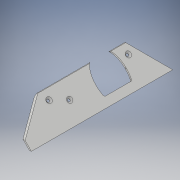
# Autodesk Inventor part: Bok2mm
Saved by Autodesk Inventor 2019 (Build 230136000, 136)
## iProperties
Created: 2022-01-23
Part Number: Bok2mm
Material: Ogólny
Document SubType Name: Modeling
Designer: Michał
Density: 1 g/cm^3
Appearance: Domyślna
Author: Michał
Autodesk Inventor part; units mm, degrees
ref_plane "YZ Plane" through (0, 0, 0) normal (1, 0, 0) x (0, 1, 0)
ref_plane "XZ Plane" through (0, 0, 0) normal (0, 1, 0) x (-1, 0, 0)
ref_plane "XY Plane" through (0, 0, 0) normal (0, 0, 1) x (1, 0, 0)
sketch "Szkic1" plane through (0, 0, 0) normal (0, 0, 1) x (1, 0, 0)
  line L0 (0, 0) -> (-30, 30)
  line L1 (-30, 30) -> (-30, 27.1716)
  line L2 (-30, 27.1716) -> (-2.8284, 0)
  line L3 (-2.8284, 0) -> (0, 0)
  line L4 (-30, 27.1716) -> (-30.8284, 28)
  line L5 (-30.8284, 28) -> (-30.8284, 30)
  line L6 (-30.8284, 30) -> (-30, 30)
  dimension "d0" = 2
  dimension "d1" = 30
  dimension "d2" = 45
  dimension "d3" = 2
  constraints: 14 end point, 2 vertical, 1 collinear, 1 horizontal, 1 parallel, 1 perpendicular
  measures "d0" distance between parallel lines of L0 L2
  measures "d1" distance from line of L3 L0.end
  measures "d2" angle of L3 L2
  measures "d3" distance of L4.end L5.end
extrude "Wyciągnięcie proste1" add sketch "Szkic1" along normal blind 180.257
sketch "Szkic2" plane through (-30.8284, 28, 0) normal (-1, 0, 0) x (0, 0, 1)
  line L0 (0, 0) -> (0, -28) projected
  line L1 (0, 2) -> (180.257, 2) projected
  line L2 (0, -28) -> (0, 2)
  line L3 (0, 2) -> (30, 2)
  line L4 (0, 0) -> (180.257, 0) projected
  line L5 (30, 2) -> (0, -28)
  line L6 (180.257, 2) -> (180.257, -20)
  line L7 (180.257, 0) -> (180.257, -28) projected
  line L8 (180.257, 2) -> (142.1519, 2)
  line L9 (180.257, -20) -> (142.1519, 2)
  dimension "d6" = 45
  dimension "d7" = 30
  dimension "d8" = 22
  constraints: 12 end point, 2 point on line, 1 parallel, 1 perpendicular
  measures "d6" angle of L5 L0
  measures "d7" angle of L1 L9
  measures "d8" distance of L1.end L6.end
extrude "Wyciągnięcie proste2" cut sketch "Szkic2" against normal through all contours L4 L5 L0 | L2 L1 L5 L4 | L9 L1 L6 L4 | L4 L6 L9
sketch "Szkic3" plane through (0, 0, 0) normal (0.7071, 0.7071, 0) x (-0.7071, 0.7071, 0)
  line L0 (42.4264, 30) -> (42.4264, 142.1519) construction
  line L1 (42.4264, 115.152) -> (23.012, 115.152) construction
  circle A0 centre (32.012, 135.152) radius 1.6
  circle A1 centre (23.012, 115.152) radius 1.6
  circle A2 centre (32.012, 33.9815) radius 1.6
  line L2 (41.598, 28) -> (41.598, 145.616) projected
  point P0 (0, 0)
  dimension "d17" = 3.2
  dimension "d37" = 9.586
  dimension "d38" = 5.9815
  dimension "d39" = 10.464
  dimension "d40" = 30.464
  dimension "d41" = 18.586
  constraints: 3 centre point, 2 coincident, 2 end point, 2 equal radius, 1 horizontal, 1 point on line, 1 vertical alignment
  measures "d17" diameter of A0
  measures "d37" distance from line of L2 A2.centre
  measures "d38" vertical distance of A2.centre L2.start
  measures "d39" vertical distance of L2.end A0.centre
  measures "d40" vertical distance of L1.end L2.end
  measures "d41" distance from line of L2 L1.end
extrude "Wyciągnięcie proste3" cut sketch "Szkic3" against normal through all
chamfer "Faza1" distance 1.85 distance2 1.75 1 edges at (-15.1406, 15.1406, 115.152) measured on face at (-5.0469, 5.0469, 98.4697)
chamfer "Faza2" distance 1.85 distance2 1.75 1 edges at (-21.5045, 21.5045, 135.152) measured on face at (-4.6108, 4.6108, 98.4697)
chamfer "Faza3" distance 1.85 distance2 1.75 1 edges at (-21.5045, 21.5045, 33.9815) measured on face at (-4.6108, 4.6108, 98.4697)
sketch "Szkic4" plane through (-30.8284, 28, 28) normal (-1, 0, 0) x (0, 0, 1)
  circle A0 centre (34.7574, -13) radius 19.25
  line L0 (-28, -28) -> (152.257, -28) projected
  dimension "d29" = 62.7574
  dimension "d30" = 38.5
  dimension "d31" = 15
  constraints: 1 centre point
  measures "d29" horizontal distance of L0.start A0.centre
  measures "d30" diameter of A0
  measures "d31" distance from line of L0 A0.centre
extrude "Wyciągnięcie proste4" cut sketch "Szkic4" against normal blind 22.5
sketch "Szkic5" plane through (0, 0, 0) normal (0.7071, 0.7071, 0) x (-0.7071, 0.7071, 0)
  line L0 (9.7782, 79.4999) -> (9.7782, 46.0149) projected
  line L1 (9.7782, 79.4999) -> (9.7782, 46.0149)
  ellipse E0 centre (16.4957, 62.7574) end of major axis (16.4957, 43.5074) minor radius 13.6118 (9.7782, 46.0149) -> (11.7782, 44.7005) ccw projected
  ellipse E1 centre (16.4957, 62.7574) end of major axis (16.4957, 43.5074) minor radius 13.6118 (11.7782, 80.8143) -> (9.7782, 79.4999) ccw projected
  ellipse E2 centre (23.2132, 62.7574) end of major axis (50.4368, 62.7574) minor radius 19.25 (41.598, 76.9547) -> (9.7782, 79.4999) ccw projected
  ellipse E3 centre (32.4056, 62.7574) end of major axis (32.4056, 43.5074) minor radius 13.6118 (43.0122, 74.8223) -> (41.598, 76.9547) ccw projected
  ellipse E4 centre (32.4056, 62.7574) end of major axis (32.4056, 43.5074) minor radius 13.6118 (41.598, 48.5601) -> (43.0122, 50.6925) ccw projected
  line L2 (43.0122, 74.8223) -> (43.0122, 50.6925)
  ellipse E5 centre (23.2132, 62.7574) end of major axis (50.4368, 62.7574) minor radius 19.25 (9.7782, 46.0149) -> (41.598, 48.5601) ccw projected
  ellipse E6 centre (21.2132, 62.7574) end of major axis (48.4368, 62.7574) minor radius 19.25 (11.7782, 44.7005) -> (42.4264, 50.6925) ccw projected
  ellipse E7 centre (21.2132, 62.7574) end of major axis (48.4368, 62.7574) minor radius 19.25 (42.4264, 74.8223) -> (11.7782, 80.8143) ccw projected
  line L3 (42.4264, 30) -> (42.4264, 50.6925) projected
  line L4 (42.4264, 74.8223) -> (42.4264, 50.6925)
  point P0 (0, 0)
  point P1 (41.598, 48.5601)
  constraints: 6 end point, 2 vertical, 1 coincident, 1 collinear, 10 other
extrude "Wyciągnięcie proste5" cut sketch "Szkic5" against normal through all
